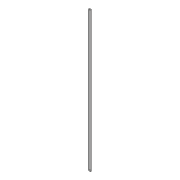
# Autodesk Inventor part: Part21
Saved by Autodesk Inventor 2017 (Build 210142000, 142)
## iProperties
Created: 2019-07-22
Part Number: Part21
Material: Generic
Document SubType Name: Modeling
Designer: Admin
Density: 1 g/cm^3
Appearance: Default
Author: Admin
Autodesk Inventor part; units mm, degrees
ref_plane "YZ Plane" through (0, 0, 0) normal (1, 0, 0) x (0, 1, 0)
ref_plane "XZ Plane" through (0, 0, 0) normal (0, 1, 0) x (-1, 0, 0)
ref_plane "XY Plane" through (0, 0, 0) normal (0, 0, 1) x (1, 0, 0)
sketch "Sketch1" plane through (0, 0, 0) normal (0, 0, 1) x (1, 0, 0)
  line L0 (0, 0) -> (-4, 0)
  line L1 (-4, 0) -> (-4, 10)
  line L2 (-4, 10) -> (0, 10)
  line L3 (0, 10) -> (0, 0)
  line L4 (-28, 0) -> (-24, 0)
  line L5 (-24, 0) -> (-24, 10)
  line L6 (-24, 10) -> (-28, 10)
  line L7 (-28, 10) -> (-28, 0)
  dimension "d0" = 4
  dimension "d1" = 10
  constraints: 16 end point, 2 parallel, 1 horizontal, 1 perpendicular
  measures "d0" distance of L1.end L2.end
  measures "d1" distance between parallel lines of L2 L0
extrude "Extrusion1" add sketch "Sketch1" along normal blind 1950
sketch "Sketch2" plane through (0, 0, 1950) normal (0, 0, 1) x (1, 0, 0)
  line L0 (-24, 10) -> (-28, 10) projected
  line L1 (-28, 10) -> (0, 10)
  line L2 (0, 10) -> (0, 0)
  line L3 (0, 0) -> (-28, 0)
  line L4 (-28, 0) -> (-28, 10)
  constraints: 8 end point, 2 parallel, 1 horizontal, 1 perpendicular
extrude "Extrusion2" add sketch "Sketch2" along normal blind 10
sketch "Sketch3" plane through (0, 0, 0) normal (0, 0, -1) x (-1, 0, 0)
  line L0 (0, 0) -> (4, 0) projected
  line L1 (0, 0) -> (28, 0)
  line L2 (28, 0) -> (28, 10)
  line L3 (28, 10) -> (0, 10)
  line L4 (0, 10) -> (0, 0)
  constraints: 8 end point, 2 parallel, 1 horizontal, 1 perpendicular
extrude "Extrusion3" add sketch "Sketch3" along normal blind 10
body "Solid1"
